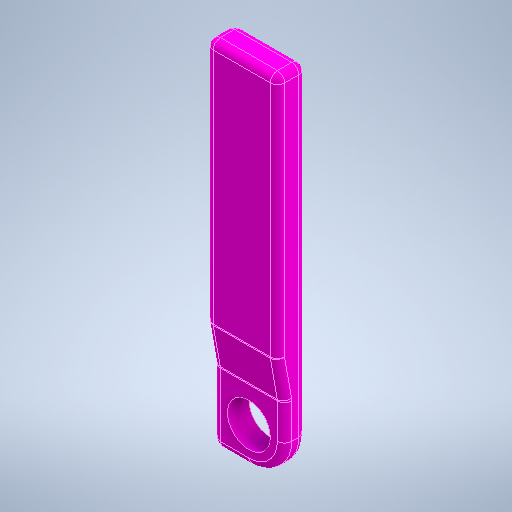
# Autodesk Inventor part: Reverse Lockout
Saved by Autodesk Inventor 2025.2 (Build 292293000, 293)
## iProperties
Created: 2025-02-09
Part Number: Reverse Lockout
Material: Generic
Document SubType Name: Modeling
Designer: eason
Density: 1 g/cm^3
Appearance: Magenta
Author: eason
Autodesk Inventor part; units mm, degrees
ref_plane "YZ Plane" through (0, 0, 0) normal (1, 0, 0) x (0, 1, 0)
ref_plane "XZ Plane" through (0, 0, 0) normal (0, 1, 0) x (-1, 0, 0)
ref_plane "XY Plane" through (0, 0, 0) normal (0, 0, 1) x (1, 0, 0)
sketch "Sketch1" plane through (0, 0, 0) normal (0, 0, 1) x (1, 0, 0)
  circle A0 centre (0, 0) radius 3
  line L0 (-5, 45) -> (5, 45)
  line L1 (5, 45) -> (5, 0)
  line L2 (0, -5) -> (-5, -5)
  line L3 (-5, -5) -> (-5, 45)
  line L4 (0, 55.2071) -> (0, -16.2426) projected
  line L5 (-7.2071, 0) -> (8.2426, 0) projected
  arc A1 (0, -5) -> (5, 0) centre (0, 0) ccw
  dimension "d0" = 6
  dimension "d1" = 10
  dimension "d2" = 50
  dimension "d3" = 5
  constraints: 8 end point, 2 centre point, 2 parallel, 2 point on circle, 2 point on line, 2 tangent, 1 coincident, 1 horizontal, 1 perpendicular
  measures "d0" diameter of A0
  measures "d1" distance between parallel lines of L1 L3
  measures "d2" distance between parallel lines of L2 L0
  measures "d3" distance between parallel lines of L2 L5
extrude "Extrusion1" add sketch "Sketch1" along normal blind 4 contours L5 A1 L4 A0 | A0 L4 L0 L1 L5 | A0 L5 L3 L0 L4 | L4 L2 L3 L5 A0
sketch "Sketch2" plane through (-5, -5, 0) normal (-1, 0, 0) x (0, 0, 1)
  line L0 (0, 0) -> (4, 0) projected
  line L1 (3, 0) -> (3, 10)
  line L2 (3, 10) -> (4, 15.6713)
  line L3 (4, 50) -> (4, 0) projected
  point P0 (0, 5)
  dimension "d6" = 1
  dimension "d7" = 10
  dimension "d8" = 10
  constraints: 4 end point, 2 point on line, 1 vertical
  measures "d6" distance between parallel lines of L3 L1
  measures "d7" angle of L3 L2
  measures "d8" distance of L1.start L1.end
extrude "Extrusion2" cut sketch "Sketch2" against normal up to surface (10 mm away)
fillet "Fillet1" radius 1 19 edges at (-5, 20, 0) (-5, 27.8356, 4) (-5, 7.8356, 3.5) (-5, 0, 3) (5, 7.8356, 3.5) (5, 27.8356, 4) (3.5355, -3.5355, 3) (-2.5, -5, 3) (5, 2.5, 3) (-5, 45, 2) (5, 45, 2) (0, 45, 4) (0, 45, 0) (3.5355, -3.5355, 0) (-2.5, -5, 0) (5, 22.5, 0) (-5, -5, 1.5) (0, 5, 3) (0, 10.6713, 4)
body "Solid1"
